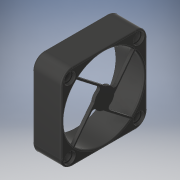
# Autodesk Inventor part: WIATRAK
Saved by Autodesk Inventor 2019.3 (Build 233278000, 278)
## iProperties
Created: 2019-11-17
Part Number: WIATRAK
Material: Ogólny
Document SubType Name: Modeling
Designer: macie
Density: 1 g/cm^3
Appearance: Domyślna
Author: macie
Autodesk Inventor part; units mm, degrees
ref_plane "YZ Plane" through (0, 0, 0) normal (1, 0, 0) x (0, 1, 0)
ref_plane "XZ Plane" through (0, 0, 0) normal (0, 1, 0) x (-1, 0, 0)
ref_plane "XY Plane" through (0, 0, 0) normal (0, 0, 1) x (1, 0, 0)
sketch "Szkic1" plane through (0, 0, 0) normal (1, 0, 0) x (0, 1, 0)
  line L0 (-15, 15) -> (15, 15)
  line L1 (15, 15) -> (15, -15)
  line L2 (15, -15) -> (-15, -15)
  line L3 (-15, -15) -> (-15, 15)
  line L4 (-15, 15) -> (15, -15) construction
  line L5 (15, 15) -> (-15, -15) construction
  line L6 (0, 0) -> (12.0208, 12.0208) construction
  circle A0 centre (12.0208, 12.0208) radius 1.5
  line L7 (0, 0) -> (0, 7.3193) construction
  line L8 (0, 0) -> (3.8373, 0) construction
  circle A1 centre (-12.0208, 12.0208) radius 1.5
  circle A2 centre (12.0208, -12.0208) radius 1.5
  circle A3 centre (-12.0208, -12.0208) radius 1.5
  circle A4 centre (0, 0) radius 14
  dimension "d0" = 30
  dimension "d1" = 30
  dimension "d2" = 17
  dimension "d3" = 3
  dimension "d4" = 28
  constraints: 18 end point, 5 centre point, 3 symmetric about line, 2 coincident, 2 horizontal, 2 midpoint, 2 parallel, 1 perpendicular, 1 point on line, 1 vertical, 3 other
  measures "d0" distance of L1.end L2.end
  measures "d1" distance of L0.end L1.end
  measures "d2" distance of L6.start L6.end
  measures "d3" diameter of A0
  measures "d4" diameter of A4
extrude "Wyciągnięcie proste1" add sketch "Szkic1" along normal blind 10
fillet "Zaokrąglenie1" radius 4 4 edges at (5, 15, 15) (5, 15, -15) (5, -15, 15) (5, -15, -15)
sketch "Szkic2" plane through (10, 0, 0) normal (1, 0, 0) x (0, 0, -1)
  circle A0 centre (0, 0) radius 3.5
  line L0 (0, 3.5) -> (-1, 3.5) construction
  line L1 (-1, 3.5) -> (1, 3.5) construction
  circle A1 centre (0, 0) radius 14 construction
  line L2 (0, 0) -> (0, 1.6463) construction
  arc A2 (-1, 3.3541) -> (-1.5597, 13.9129) centre (-31.1594, 7.0497) ccw
  arc A3 (1.5597, 13.9129) -> (1, 3.3541) centre (31.1594, 7.0497) ccw
  arc A4 (1.5597, 13.9129) -> (-1.5597, 13.9129) centre (0, 0) ccw
  dimension "d8" = 7
  dimension "d9" = 1
  dimension "d10" = 2
  constraints: 11 point on circle, 6 end point, 4 centre point, 3 symmetric about line, 1 coincident, 1 concentric, 1 horizontal, 1 point on line, 1 tangent, 1 vertical, 1 other
  measures "d8" diameter of A0
  measures "d9" distance of L0.start L0.end
  measures "d10" distance of L0.end L1.end
extrude "Wyciągnięcie proste2" add sketch "Szkic2" against normal blind 1 contours A0
sketch "Szkic3" plane through (10, 0, 0) normal (1, 0, 0) x (0, 0, -1)
  arc A0 (0.3871, 3.4785) -> (-0.53, 3.4596) centre (0, 0) ccw
  arc A1 (-9.0021, 10.722) -> (-9.443, 10.3358) centre (0, 0) ccw
  circle A2 centre (0, 0) radius 3.5 projected
  line L0 (-0.53, 3.4596) -> (-9.443, 10.3358)
  circle A3 centre (0, 0) radius 14 projected
  line L1 (0.3871, 3.4785) -> (-9.0021, 10.722)
  constraints: 4 end point, 4 point on circle, 2 centre point, 2 coincident, 1 parallel, 4 other
extrude "Wyciągnięcie proste3" add sketch "Szkic3" against normal blind 1 contours A0 L0 A1 L1
pattern_circular "Szyk kołowy1" count 4 over 360 about axis through (10, 0, 0) along (-1, 0, 0) of "Wyciągnięcie proste3"
fillet "Zaokrąglenie2" radius 1 4 edges at (9.5, 3.4596, 0.53) (9.5, 0.53, -3.4596) (9.5, -0.53, 3.4596) (9.5, -3.4596, -0.53)
fillet "Zaokrąglenie3" radius 0.5 16 edges at (10, -13.8284, 13.8284) (10, -15, 0) (10, -13.8284, -13.8284) (10, 0, -15) (10, 13.8284, -13.8284) (10, 15, 0) (10, 13.8284, 13.8284) (10, 0, 15) (0, 13.8284, 13.8284) (0, 15, 0) (0, 13.8284, -13.8284) (0, 0, -15) (0, -13.8284, -13.8284) (0, -15, 0) (0, -13.8284, 13.8284) (0, 0, 15)
fillet "Zaokrąglenie4" radius 0.5 5 edges at (10, -13.9695, 0.9239) (10, -0.9239, -13.9695) (10, 12.8102, -5.6479) (10, 13.155, 4.7902) (10, 0.9239, 13.9695)
sketch "Szkic4" plane through (10, 0, 0) normal (1, 0, 0) x (0, 0, -1)
  circle A0 centre (-12.0208, 12.0208) radius 1.5 projected
  circle A1 centre (-12.0208, 12.0208) radius 2
  circle A2 centre (12.0208, 12.0208) radius 1.5 projected
  circle A3 centre (12.0208, 12.0208) radius 2
  circle A4 centre (12.0208, -12.0208) radius 1.5 projected
  circle A5 centre (12.0208, -12.0208) radius 2
  circle A6 centre (-12.0208, -12.0208) radius 1.5 projected
  circle A7 centre (-12.0208, -12.0208) radius 2
  point P0 (0, 0)
  dimension "d21" = 4
  dimension "d22" = 4
  dimension "d23" = 4
  dimension "d24" = 4
  constraints: 4 centre point, 4 coincident
  measures "d21" diameter of A1
  measures "d22" diameter of A3
  measures "d23" diameter of A5
  measures "d24" diameter of A7
extrude "Wyciągnięcie proste4" cut sketch "Szkic4" against normal blind 1
